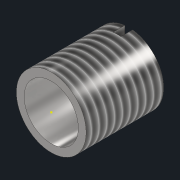
# Autodesk Inventor part: rod330_end_screw
Saved by Autodesk Inventor 2022 (Build 260153000, 153)
## iProperties
Created: 2024-03-31
Part Number: rod330_end_screw
Material: ステンレス鋼
Document SubType Name: Modeling
Designer: gisen
Mass: 24.9491 g
Surface Area: 22.8814 cm^2
Volume: 3.11864 cm^3
Density: 8 g/cm^3
Appearance: 半つや出し
Author: gisen
Autodesk Inventor part; units mm, degrees
ref_plane "YZ Plane" through (0, 0, 0) normal (1, 0, 0) x (0, 1, 0)
ref_plane "XZ Plane" through (0, 0, 0) normal (0, 1, 0) x (-1, 0, 0)
ref_plane "XY Plane" through (0, 0, 0) normal (0, 0, 1) x (1, 0, 0)
sketch "スケッチ1" plane through (0, 0, 0) normal (0, 0, 1) x (1, 0, 0)
  circle A0 centre (0, 0) radius 9
  circle A1 centre (0, 0) radius 1
  dimension "d0" = 18
  dimension "d3" = 2
  constraints: 2 centre point, 2 coincident
  measures "d0" diameter of A0
  measures "d3" diameter of A1
extrude "押し出し1" add sketch "スケッチ1" along normal mid plane 20
sketch "スケッチ2" plane through (0, 0, -10) normal (0, 0, -1) x (-1, 0, 0)
  line L0 (-1, 10.2383) -> (1, 10.2383)
  line L1 (1, 10.2383) -> (1, -10.4548)
  line L2 (1, -10.4548) -> (-1, -10.4548)
  line L3 (-1, -10.4548) -> (-1, 10.2383)
  point P0 (0, 0)
  point P1 (0, -10.4548)
  dimension "d4" = 2
  constraints: 8 end point, 2 parallel, 1 horizontal, 1 midpoint, 1 perpendicular, 1 vertical alignment
  measures "d4" distance of L0.start L0.end
extrude "押し出し2" cut sketch "スケッチ2" against normal blind 3
thread "ねじ1" size "M20x2" class "6g" standard "ISO Metric profile" full length
sketch "スケッチ3" plane through (0, 0, 10) normal (0, 0, 1) x (1, 0, 0)
  point P0 (0, 0)
sketch "スケッチ4" plane through (0, 0, 10) normal (0, 0, 1) x (1, 0, 0)
  circle A0 centre (0, 0) radius 7
  dimension "d9" = 14
  constraints: 1 centre point, 1 coincident
  measures "d9" diameter of A0
extrude "押し出し3" cut sketch "スケッチ4" against normal blind 12
